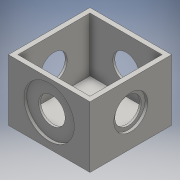
# Autodesk Inventor part: sampleChamber_singlePiece_filipeSample_V1
Saved by Autodesk Inventor 2016 (Build 200138000, 138)
## iProperties
Created: 2016-07-14
Part Number: sampleChamber_singlePiece_filipeSample_V1
Material: Generic
Document SubType Name: Modeling
Designer: sims01
Density: 1 g/cm^3
Appearance: Default
Author: sims01
Autodesk Inventor part; units mm, degrees
ref_plane "YZ Plane" through (0, 0, 0) normal (1, 0, 0) x (0, 1, 0)
ref_plane "XZ Plane" through (0, 0, 0) normal (0, 1, 0) x (-1, 0, 0)
ref_plane "XY Plane" through (0, 0, 0) normal (0, 0, 1) x (1, 0, 0)
sketch "Sketch1" plane through (0, 0, 0) normal (0, 0, 1) x (1, 0, 0)
  line L0 (-30, 30) -> (30, 30)
  line L1 (30, 30) -> (30, -30)
  line L2 (30, -30) -> (-30, -30)
  line L3 (-30, -30) -> (-30, 30)
  point P0 (0, 0)
  dimension "d0" = 60
  dimension "d1" = 60
  dimension "d2" = 30
  dimension "d3" = 30
  constraints: 8 end point, 2 parallel, 1 horizontal, 1 perpendicular
  measures "d0" distance of L0.start L0.end
  measures "d1" distance of L2.end L0.start
  measures "d2" distance from line of point (0, 0) L1
  measures "d3" distance from line of point (0, 0) L0
extrude "Extrusion1" add sketch "Sketch1" along normal blind 5
sketch "Sketch2" plane through (0, 0, 5) normal (0, 0, 1) x (1, 0, 0)
  line L0 (-26.5, 26.5) -> (26.5, 26.5)
  line L1 (26.5, 26.5) -> (26.5, -26.5)
  line L2 (26.5, -26.5) -> (-26.5, -26.5)
  line L3 (-26.5, -26.5) -> (-26.5, 26.5)
  line L4 (30, 30) -> (-30, 30) projected
  line L5 (30, -30) -> (30, 30) projected
  line L6 (-30, 30) -> (30, 30)
  line L7 (30, 30) -> (30, -30)
  line L8 (30, -30) -> (-30, -30)
  line L9 (-30, -30) -> (-30, 30)
  point P0 (0, 0)
  dimension "d6" = 53
  dimension "d7" = 53
  dimension "d8" = 26.5
  dimension "d9" = 26.5
  constraints: 16 end point, 4 parallel, 2 horizontal, 2 perpendicular
  measures "d6" distance of L0.start L0.end
  measures "d7" distance of L0.end L1.end
  measures "d8" distance from line of point (0, 0) L0
  measures "d9" distance from line of point (0, 0) L1
extrude "Extrusion2" add sketch "Sketch2" along normal blind 40
sketch "Sketch3" plane through (-30, -30, 0) normal (0, -1, 0) x (1, 0, 0)
  circle A0 centre (30, 23.5) radius 18.5
  point P0 (30, 0)
  dimension "d12" = 37
  dimension "d13" = 23.5
  constraints: 1 centre point
  measures "d12" diameter of A0
  measures "d13" distance of point (30, 0) A0.centre
extrude "Extrusion3" cut sketch "Sketch3" against normal blind 2
sketch "Sketch4" plane through (0, -28, 23.5) normal (0, -1, 0) x (1, 0, 0)
  circle A0 centre (0, 0) radius 9.75
  circle A1 centre (0, 0) radius 18.5 projected
  point P0 (0, -23.5)
  dimension "d19" = 19.5
  constraints: 1 centre point, 1 concentric
  measures "d19" diameter of A0
extrude "Extrusion4" cut sketch "Sketch4" against normal blind 2 contours A0
pattern_circular "Circular Pattern2" count 4 over 360 about axis through (0, 0, -10) along (0, 0, 1) of "Extrusion4"
mirror "Mirror1" about plane through (0, 0, 0) normal (0, 1, 0) of "Extrusion3"
sketch "Sketch6" plane through (30, -30, 0) normal (1, 0, 0) x (0, 0, -1)
  circle A0 centre (-23.5, 30) radius 12.5
  circle A1 centre (-23.5, 30) radius 9.75 projected
  point P0 (0, 30)
  dimension "d28" = 25
  constraints: 1 centre point, 1 concentric
  measures "d28" diameter of A0
extrude "Extrusion6" cut sketch "Sketch6" against normal blind 2 contours A0 | A1
mirror "Mirror2" about plane through (0, 0, 0) normal (1, 0, 0) of "Extrusion6"
equation "\"d2\" = 0.5 * d0"
equation "\"d3\" = 0.5 * d1"
equation "\"d8\" = 0.5 * d7"
equation "\"d9\" = 0.5 * d6"
body "Solid1"
